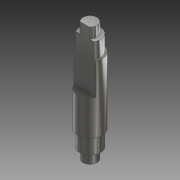
# Autodesk Inventor part: 2nd_phalanx_shaft
Saved by Autodesk Inventor 2017 SP1 (Build 210196100, 196)
## iProperties
Created: 2017-06-05
Part Number: 2nd_phalanx_shaft
Material: Generic
Document SubType Name: Modeling
Designer: Tomasz
Density: 1 g/cm^3
Appearance: Steel - Polished
Author: Tomasz
Autodesk Inventor part; units mm, degrees
ref_plane "YZ Plane" through (0, 0, 0) normal (1, 0, 0) x (0, 1, 0)
ref_plane "XY Plane" through (0, 0, 0) normal (0, 0, 1) x (1, 0, 0)
sketch "Sketch1" plane through (0, 0, 0) normal (0, 1, 0) x (-1, 0, 0)
  line L0 (0, 18.1135) -> (0, -15.5197) construction
  line L1 (0, 0) -> (5.9379, 0) construction
  line L2 (0, -8.5) -> (1, -8.5)
  line L3 (1, -8.5) -> (1, -7)
  line L4 (1, -7) -> (1.1561, -7)
  line L5 (1.5, -4.75) -> (1.75, -4.75)
  line L6 (1.75, -4.75) -> (1.75, 4.75)
  line L7 (1.75, 4.75) -> (1.5, 4.75)
  line L8 (1.5, 4.75) -> (1.5, 7)
  line L9 (1.5, 7) -> (1, 7)
  line L10 (1, 7) -> (1, 8.5)
  line L11 (1, 8.5) -> (0, 8.5)
  line L12 (0, -8.5) -> (0, 8.5)
  line L13 (1.5, -4.75) -> (1.5, -7)
  line L14 (1.5, -7) -> (1.1561, -7)
  dimension "d7" = 17
  dimension "d9" = 1
  dimension "d10" = 1.5
  dimension "d11" = 14
  dimension "d12" = 1.75
  dimension "d13" = 9.5
  constraints: 30 end point, 7 perpendicular, 6 point on line, 2 horizontal, 2 vertical, 1 collinear, 3 other
  measures "d7" distance between parallel lines of L11 L2
  measures "d9" distance between parallel lines of L0 L10
  measures "d10" distance between parallel lines of L8 L0
  measures "d11" distance between parallel lines of L14 L9
  measures "d12" distance between parallel lines of L6 L12
  measures "d13" distance between parallel lines of L7 L5
revolve "Revolution1" add sketch "Sketch1" angle 360 about axis through (0, 0, 18.1135) along (0, 0, -1)
ref_plane "Work Plane1" through (0, -1.75, 0) normal (0, 1, 0) x (-1, 0, 0)
sketch "Sketch2" plane through (0, -1.75, 0) normal (0, 1, 0) x (-1, 0, 0)
  line L0 (-1.75, -4.75) -> (1.75, -4.75) projected
  line L1 (-1.75, 4.75) -> (1.75, 4.75) projected
  line L2 (-1.75, -4.75) -> (1.75, -4.75) projected
  line L3 (-1.75, 4.75) -> (-1.75, -4.75) projected
  line L4 (1.75, 4.75) -> (1.75, -4.75) projected
  line L5 (-1.75, 0.25) -> (1.75, 0.25)
  line L6 (1.75, 0.25) -> (1.75, 8.5)
  line L7 (-1.75, 8.5) -> (-1.75, 0.25)
  line L8 (-1.5, 7) -> (1.5, 7) projected
  line L9 (-1.5, 4.75) -> (1.5, 4.75) projected
  line L10 (-1, 8.5) -> (1, 8.5) projected
  line L11 (-1.75, 8.5) -> (1.75, 8.5)
  dimension "d17" = 4.5
  constraints: 8 end point, 3 point on line, 2 horizontal, 1 parallel, 1 perpendicular, 1 vertical
  measures "d17" distance between parallel lines of L5 L1
extrude "Extrusion1" cut sketch "Sketch2" along normal blind 1 contours L3 L1 L4 L5 | L7 L11 L10 L6 L1
body "Solid1"
